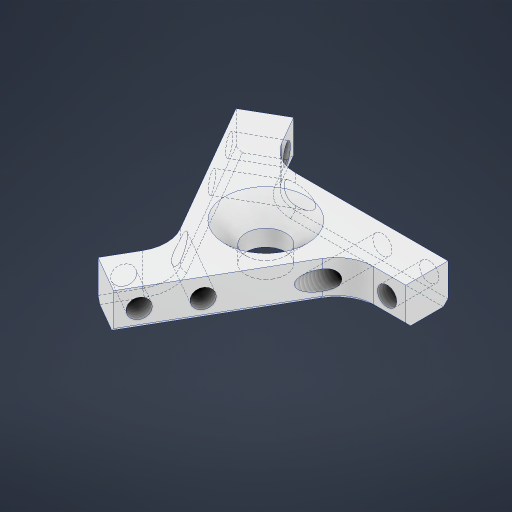
# Autodesk Inventor part: ServoCap V2
Saved by Autodesk Inventor 2023 (Build 270158000, 158)
## iProperties
Created: 2023-02-26
Part Number: ServoCap V2
Material: Aluminum 6061
Document SubType Name: Modeling
Designer: roota
Density: 2.7 g/cm^3
Appearance: Aluminum - Flat
Author: roota
Autodesk Inventor part; units mm, degrees
ref_plane "YZ Plane" through (0, 0, 0) normal (1, 0, 0) x (0, 1, 0)
ref_plane "XZ Plane" through (0, 0, 0) normal (0, 1, 0) x (-1, 0, 0)
ref_plane "XY Plane" through (0, 0, 0) normal (0, 0, 1) x (1, 0, 0)
sketch "Sketch1" plane through (0, 0, 0) normal (0, 1, 0) x (-1, 0, 0)
  circle A0 centre (0, 0) radius 11.9 construction
  line L0 (0, -11.9) -> (-27, -11.9)
  line L1 (-27, -11.9) -> (-27, -2.9)
  line L2 (-27, -2.9) -> (0, -2.9)
  line L3 (0, -2.9) -> (0, -11.9)
  line L4 (10.3057, 5.95) -> (23.8057, -17.4327)
  line L5 (23.8057, -17.4327) -> (16.0115, -21.9327)
  line L6 (16.0115, -21.9327) -> (2.5115, 1.45)
  line L7 (2.5115, 1.45) -> (10.3057, 5.95)
  line L8 (-10.3057, 5.95) -> (3.1943, 29.3327)
  line L9 (3.1943, 29.3327) -> (10.9885, 24.8327)
  line L10 (10.9885, 24.8327) -> (-2.5115, 1.45)
  line L11 (-2.5115, 1.45) -> (-10.3057, 5.95)
  line L12 (-10.3057, 5.95) -> (-15.4153, -2.9)
  line L13 (10.3057, 5.95) -> (5.1962, 14.8)
  line L14 (0, -11.9) -> (10.2191, -11.9)
  dimension "d2" = 360
  dimension "d5" = 27
  dimension "d6" = 9
  dimension "d7" = 11.9
  constraints: 30 end point, 4 point on line, 2 collinear, 2 parallel, 2 vertical alignment, 1 coincident, 1 horizontal, 1 perpendicular, 27 other
  measures "d5" distance from line of point (0, 0) L1
  measures "d6" distance of L0.end L1.end
  measures "d7" distance from line of point (0, 0) L0
extrude "Extrusion1" add sketch "Sketch1" along normal blind 8
sketch "Sketch2" plane through (0, 8, 0) normal (0, 1, 0) x (1, 0, 0)
  circle A0 centre (0, 0) radius 4.25
  dimension "d10" = 8.5
  constraints: 1 centre point, 1 coincident
  measures "d10" diameter of A0
extrude "Extrusion2" cut sketch "Sketch2" against normal blind 8
chamfer "Chamfer1" distance 4.5 angle 45 1 edges at (-4.25, 8, 0)
fillet "Fillet1" radius 8 3 edges at (15.4153, 4, -2.9) (-5.1962, 4, 14.8) (-10.2191, 4, -11.9)
sketch "Sketch3" plane through (-3.1943, 0, 29.3327) normal (0.8660254, 0, 0.5) x (0.5, 0, -0.8660254)
  circle A0 centre (4, 4) radius 2.5
  circle A1 centre (14, 4) radius 2.5
  line L0 (0, 0) -> (0, 8) projected
  line L1 (0, 0) -> (32.6003, 0) projected
  point P0 (27, 0)
  dimension "d17" = 10
  dimension "d18" = 4
  dimension "d19" = 4
  dimension "d20" = 5
  constraints: 2 centre point, 1 equal radius, 1 horizontal alignment
  measures "d17" distance of A0.centre A1.centre
  measures "d18" distance from line of L0 A0.centre
  measures "d19" distance from line of A0.centre L1
  measures "d20" diameter of A1
hole "Hole1" at (-1.1943, 4, 25.8686) at (3.8057, 4, 17.2083) direction (-0.8660254, 0, -0.5) diameter 4.134 end through all thread size "M5x0.8" class "6H" standard "ISO Metric profile"
pattern_circular "Circular Pattern1" count 3 over 360 about axis through (0, 8, 0) along (0, -1, 0) of "Hole1"
chamfer "Chamfer3" distance 1 angle 45 9 edges at (4.9558, 0, 15.2163) (16.0341, 0, -1.8282) (23.517, 0, -2.9) (-9.247, 0, 21.8163) (-6.4338, 0, 14.8) (-15.6556, 0, -3.3163) (10.6999, 0, -11.9) (-9.6003, 0, -12.9718) (-14.27, 0, -18.9163)
body "Solid1"
